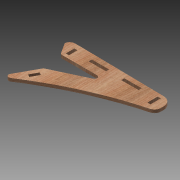
# Autodesk Inventor part: Pata con lado2
Saved by Autodesk Inventor 2015 (Build 190159000, 159)
## iProperties
Created: 2016-02-08
Part Number: Pata con lado2
Material: Wood (Birch)
Document SubType Name: Modeling
Designer: iberopuebla
Density: 0.55 g/cm^3
Appearance: Birch - Natural Polished
Author: iberopuebla
Autodesk Inventor part; units mm, degrees
ref_plane "YZ Plane" through (0, 0, 0) normal (1, 0, 0) x (0, 1, 0)
ref_plane "XZ Plane" through (0, 0, 0) normal (0, 1, 0) x (-1, 0, 0)
ref_plane "XY Plane" through (0, 0, 0) normal (0, 0, 1) x (1, 0, 0)
sketch "Sketch1" plane through (0, 0, 0) normal (0, 0, 1) x (1, 0, 0)
  arc A0 (581.4844, 252.6536) -> (22.0836, 3.3874) centre (1090.7043, -1642.4666) ccw
  line L0 (55.6223, 267.588) -> (258.6014, 267.588)
  line L1 (264.9525, 238.9989) -> (73.5785, 149.5573)
  line L2 (5.59, 332.9002) -> (42.9906, 274.4986)
  line L3 (66.787, 143.1982) -> (0.7725, 23.1982)
  arc A1 (264.9525, 238.9989) -> (258.6014, 267.588) centre (258.6014, 252.588) ccw
  arc A2 (42.9906, 274.4986) -> (55.6223, 267.588) centre (55.6223, 282.588) ccw
  arc A3 (73.5785, 149.5573) -> (66.787, 143.1982) centre (79.9296, 135.9682) ccw
  arc A4 (0.7725, 23.1982) -> (22.0836, 3.3874) centre (13.9151, 15.9682) ccw
  arc A5 (581.4844, 252.6536) -> (607.402, 286.4547) centre (572.402, 286.4547) ccw
  line L4 (77.4986, 363.1761) -> (556.5067, 355.4189)
  arc A6 (607.402, 303.6927) -> (556.5067, 355.4189) centre (555.6691, 303.6927) ccw
  line L5 (607.402, 303.6927) -> (607.402, 286.4547)
  line L6 (34.6831, 363.1761) -> (77.4986, 363.1761)
  arc A7 (34.6831, 363.1761) -> (4.8241, 336.0808) centre (34.6831, 333.1761) ccw
  arc A8 (4.8241, 336.0808) -> (5.59, 332.9002) centre (9.8006, 335.5967) ccw
  line L7 (540.6073, 347.6664) -> (560.6073, 347.6664)
  line L8 (560.6073, 347.6664) -> (560.6073, 267.6664)
  line L9 (560.6073, 267.6664) -> (540.6073, 267.6664)
  line L10 (540.6073, 267.6664) -> (540.6073, 347.6664)
  line L11 (60.6073, 346.8815) -> (80.6073, 346.8815)
  line L12 (80.6073, 346.8815) -> (80.6073, 276.8815)
  line L13 (80.6073, 276.8815) -> (60.6073, 276.8815)
  line L14 (60.6073, 276.8815) -> (60.6073, 346.8815)
  line L15 (48.4231, 57.1621) -> (96.6231, 144.7792)
  line L16 (96.6231, 144.7792) -> (114.1465, 135.1392)
  line L17 (114.1465, 135.1392) -> (65.9465, 47.5221)
  line L18 (65.9465, 47.5221) -> (48.4231, 57.1621)
  line L19 (60.6073, 470.6868) -> (560.6073, 470.6868)
  line L20 (560.6073, 470.6868) -> (560.6073, 450.6868)
  line L21 (560.6073, 450.6868) -> (60.6073, 450.6868)
  line L22 (60.6073, 450.6868) -> (60.6073, 470.6868)
  line L23 (656.5696, 347.2322) -> (-473.2183, 347.2322) construction
  point P0 (0, 0)
  point P1 (-29.0079, -30.9362)
  point P2 (47.4161, 267.588)
  point P3 (69.1456, 147.4855)
  point P4 (622.6529, 263.2389)
  dimension "d5" = 15
  dimension "d9" = 35
  dimension "d13" = 120
  dimension "d18" = 30
  dimension "d19" = 5
  dimension "d22" = 607.402
  dimension "d27" = 20
  dimension "d28" = 80
  dimension "d29" = 20
  dimension "d30" = 70
  dimension "d33" = 20
  dimension "d35" = 20
  dimension "d36" = 100
  dimension "d39" = 500
  dimension "d40" = 20
  dimension "d41" = 500
  constraints: 48 end point, 20 point on circle, 15 tangent, 9 centre point, 8 parallel, 6 point on line, 5 horizontal, 5 perpendicular, 2 equal radius
  measures "d5" radius of A1
  measures "d9" radius of A5
  measures "d13" vertical distance of L3.start L3.end
  measures "d18" radius of A7
  measures "d19" radius of A8
  measures "d22" distance from line of L5 point (0, 0)
  measures "d27" distance of L8.end L9.end
  measures "d28" distance of L7.end L8.end
  measures "d29" distance of L12.end L13.end
  measures "d30" distance of L11.end L12.end
  measures "d33" distance of L15.end L16.end
  measures "d35" distance of L17.end L15.start
  measures "d36" distance of L15.start L15.end
  measures "d39" distance of L20.end L21.end
  measures "d40" distance of L19.end L20.end
  measures "d41" distance between parallel lines of L8 L14
extrude "Extrusion1" add sketch "Sketch1" along normal blind 18 contours A0 A4 L3 A3 L1 A1 L0 A2 L2 A8 A7 L6 L4 A6 L5 A5 | L7 L8 L9 L10 | L11 L12 L13 L14 | L15 L16 L17 L18
sketch "Sketch2" plane through (0, 0, 18) normal (0, 0, 1) x (1, 0, 0)
  line L0 (76.9002, 336.193) -> (58.9002, 336.193)
  line L1 (58.9002, 336.193) -> (58.9002, 286.193)
  line L2 (58.9002, 286.193) -> (76.9002, 286.193)
  line L3 (76.9002, 286.193) -> (76.9002, 336.193)
  line L4 (540.9002, 336.193) -> (558.9002, 336.193)
  line L5 (558.9002, 336.193) -> (558.9002, 276.193)
  line L6 (558.9002, 276.193) -> (540.9002, 276.193)
  line L7 (540.9002, 276.193) -> (540.9002, 336.193)
  line L8 (79.0927, 115.5231) -> (94.8638, 106.8471)
  line L9 (54.9927, 71.7145) -> (70.7638, 63.0385)
  line L10 (70.7638, 63.0385) -> (94.8638, 106.8471)
  line L11 (54.9927, 71.7145) -> (79.0927, 115.5231)
  line L12 (9.0599, 336.193) -> (647.4361, 336.193) construction
  point P0 (0, 0)
  point P1 (67.9002, 346.193)
  dimension "d73" = 50
  dimension "d75" = 60
  dimension "d113" = 18
  dimension "d114" = 18
  dimension "d115" = 18
  dimension "d116" = 50
  constraints: 26 end point, 4 horizontal, 4 parallel, 4 perpendicular, 1 point on line
  measures "d73" distance of L1.end L0.end
  measures "d75" distance of L4.end L5.end
  measures "d113" distance between parallel lines of L3 L1
  measures "d114" distance between parallel lines of L5 L7
  measures "d115" distance between parallel lines of L10 L11
  measures "d116" distance between parallel lines of L8 L9
extrude "Extrusion2" cut sketch "Sketch2" against normal blind 18
sketch "Sketch4" plane through (0, 0, 18) normal (0, 0, 1) x (1, 0, 0)
  line L0 (58.9002, 336.193) -> (60.0316, 335.0616)
  line L1 (58.9002, 336.193) -> (60.5002, 336.193) construction
  line L2 (76.9002, 336.193) -> (75.7688, 335.0616)
  line L3 (58.9002, 286.193) -> (60.0316, 287.3243)
  line L4 (76.9002, 286.193) -> (75.7688, 287.3243)
  circle A0 centre (60.0316, 335.0616) radius 1.6
  circle A1 centre (75.7688, 335.0616) radius 1.6
  circle A2 centre (60.0316, 287.3243) radius 1.6
  circle A3 centre (75.7688, 287.3243) radius 1.6
  line L5 (79.0927, 115.5231) -> (79.5387, 113.9865)
  line L6 (54.9927, 71.7145) -> (79.0927, 115.5231) projected
  line L7 (94.8638, 106.8471) -> (93.3272, 106.4011)
  line L8 (70.7638, 63.0385) -> (70.3178, 64.5751)
  line L9 (54.9927, 71.7145) -> (56.5293, 72.1604)
  line L10 (94.8638, 106.8471) -> (79.0927, 115.5231) projected
  circle A4 centre (79.5387, 113.9865) radius 1.6
  circle A5 centre (93.3272, 106.4011) radius 1.6
  circle A6 centre (70.3178, 64.5751) radius 1.6
  circle A7 centre (56.5293, 72.1604) radius 1.6
  line L11 (540.9002, 336.193) -> (542.0316, 335.0616)
  line L12 (558.9002, 336.193) -> (557.7688, 335.0616)
  line L13 (540.9002, 276.193) -> (542.0316, 277.3243)
  line L14 (558.9002, 276.193) -> (557.7688, 277.3243)
  circle A8 centre (542.0316, 335.0616) radius 1.6
  circle A9 centre (557.7688, 335.0616) radius 1.6
  circle A10 centre (542.0316, 277.3243) radius 1.6
  circle A11 centre (557.7688, 277.3243) radius 1.6
  point P0 (0, 0)
  dimension "d80" = 1.6
  dimension "d81" = 45
  dimension "d84" = 1.6
  dimension "d85" = 1.6
  dimension "d86" = 1.6
  dimension "d88" = 3.2
  dimension "d89" = 3.2
  dimension "d90" = 3.2
  dimension "d91" = 3.2
  dimension "d92" = 1.6
  dimension "d93" = 45
  dimension "d94" = 1.6
  dimension "d95" = 1.6
  dimension "d96" = 1.6
  dimension "d97" = 45
  dimension "d98" = 45
  dimension "d99" = 3.2
  dimension "d100" = 3.2
  dimension "d101" = 3.2
  dimension "d102" = 3.2
  dimension "d103" = 1.6
  dimension "d104" = 1.6
  dimension "d106" = 1.6
  dimension "d107" = 3.2
  dimension "d108" = 3.2
  dimension "d109" = 3.2
  dimension "d110" = 3.2
  constraints: 26 end point, 12 centre point, 10 coincident, 4 perpendicular, 2 point on line, 1 equal length, 1 horizontal
  measures "d80" distance of L0.start L0.end
  measures "d81" angle of L0 L1
  measures "d84" distance of L2.start L2.end
  measures "d85" distance of L3.start L3.end
  measures "d86" distance of L4.start L4.end
  measures "d88" diameter of A0
  measures "d89" diameter of A1
  measures "d90" diameter of A2
  measures "d91" diameter of A3
  measures "d92" distance of L5.start L5.end
  measures "d93" angle of L5 L6
  measures "d94" distance of L7.start L7.end
  measures "d95" distance of L8.start L8.end
  measures "d96" distance of L6.start L9.end
  measures "d97" angle of L9 L6
  measures "d98" angle of L10 L7
  measures "d99" diameter of A4
  measures "d100" diameter of A5
  measures "d101" diameter of A6
  measures "d102" diameter of A7
  measures "d103" distance of L11.start L11.end
  measures "d104" distance of L12.start L12.end
  measures "d106" distance of L13.start L13.end
  measures "d107" diameter of A8
  measures "d108" diameter of A9
  measures "d109" diameter of A10
  measures "d110" diameter of A11
extrude "Extrusion4" cut sketch "Sketch4" against normal blind 20
sketch "Sketch5" plane through (0, 0, 18) normal (0, 0, 1) x (1, 0, 0)
  line L0 (76.9002, 276.193) -> (58.9002, 276.193)
  line L1 (58.9002, 276.193) -> (58.9002, 346.193)
  line L2 (58.9002, 346.193) -> (76.9002, 346.193)
  line L3 (76.9002, 346.193) -> (76.9002, 276.193)
  line L4 (61.163, 336.193) -> (74.6375, 336.193) projected
  line L5 (558.9002, 346.193) -> (540.9002, 346.193)
  line L6 (540.9002, 346.193) -> (540.9002, 266.193)
  line L7 (540.9002, 266.193) -> (558.9002, 266.193)
  line L8 (558.9002, 266.193) -> (558.9002, 346.193)
  line L9 (543.163, 336.193) -> (556.6375, 336.193) projected
  line L10 (-10.8781, 346.193) -> (731.1552, 346.193) construction
  line L11 (540.9002, 333.9302) -> (540.9002, 278.4557) projected
  line L12 (76.9002, 331.193) -> (540.9002, 331.193)
  line L13 (540.9002, 331.193) -> (540.9002, 313.193)
  line L14 (540.9002, 313.193) -> (76.9002, 313.193)
  line L15 (76.9002, 313.193) -> (76.9002, 331.193)
  line L16 (164.9002, 331.193) -> (164.9002, 313.193)
  line L17 (264.9002, 331.193) -> (264.9002, 313.193)
  line L18 (352.9002, 331.193) -> (352.9002, 313.193)
  line L19 (452.9002, 331.193) -> (452.9002, 313.193)
  point P0 (0, 0)
  dimension "d117" = 70
  dimension "d118" = 10
  dimension "d119" = 80
  dimension "d120" = 10
  dimension "d121" = 18
  dimension "d122" = 15
  dimension "d123" = 464
  dimension "d124" = 100
  dimension "d125" = 100
  dimension "d128" = 88
  dimension "d129" = 88
  constraints: 34 end point, 10 point on line, 7 perpendicular, 6 parallel, 5 horizontal
  measures "d117" distance of L0.end L1.end
  measures "d118" distance between parallel lines of L4 L2
  measures "d119" distance of L6.end L5.end
  measures "d120" distance between parallel lines of L9 L5
  measures "d121" distance of L12.end L13.end
  measures "d122" distance between parallel lines of L12 L10
  measures "d123" distance of L12.start L12.end
  measures "d124" distance between parallel lines of L16 L17
  measures "d125" distance between parallel lines of L19 L18
  measures "d128" distance between parallel lines of L3 L16
  measures "d129" distance between parallel lines of L13 L19
extrude "Extrusion5" cut sketch "Sketch5" against normal blind 18 contours L16 L12 L17 L14 | L18 L12 L19 L14
sketch "Sketch6" plane through (0, 0, 18) normal (0, 0, 1) x (1, 0, 0)
  line L0 (164.9002, 331.193) -> (166.0316, 330.0616)
  line L1 (164.9002, 331.193) -> (166.5002, 331.193) construction
  line L2 (164.9002, 313.193) -> (166.0316, 314.3243)
  line L3 (264.9002, 313.193) -> (263.7688, 314.3243)
  line L4 (264.9002, 331.193) -> (263.7688, 330.0616)
  circle A0 centre (166.0316, 314.3243) radius 1.6
  circle A1 centre (166.0316, 330.0616) radius 1.6
  circle A2 centre (263.7688, 330.0616) radius 1.6
  circle A3 centre (263.7688, 314.3243) radius 1.6
  line L5 (352.9002, 331.193) -> (354.0316, 330.0616)
  line L6 (352.9002, 331.193) -> (354.5002, 331.193) construction
  line L7 (352.9002, 313.193) -> (354.0316, 314.3243)
  line L8 (452.9002, 313.193) -> (451.7688, 314.3243)
  line L9 (452.9002, 331.193) -> (451.7688, 330.0616)
  circle A4 centre (451.7688, 330.0616) radius 1.6
  circle A5 centre (451.7688, 314.3243) radius 1.6
  circle A6 centre (354.0316, 330.0616) radius 1.6
  circle A7 centre (354.0316, 314.3243) radius 1.6
  point P0 (0, 0)
  dimension "d132" = 1.6
  dimension "d133" = 45
  dimension "d134" = 3.2
  dimension "d135" = 3.2
  dimension "d136" = 3.2
  dimension "d137" = 3.2
  dimension "d138" = 1.6
  dimension "d139" = 45
  dimension "d140" = 3.2
  dimension "d141" = 3.2
  dimension "d142" = 3.2
  dimension "d144" = 3.2
  constraints: 20 end point, 8 centre point, 8 coincident, 6 perpendicular, 2 equal length, 2 horizontal
  measures "d132" distance of L0.start L0.end
  measures "d133" angle of L0 L1
  measures "d134" diameter of A0
  measures "d135" diameter of A1
  measures "d136" diameter of A2
  measures "d137" diameter of A3
  measures "d138" distance of L5.start L5.end
  measures "d139" angle of L5 L6
  measures "d140" diameter of A4
  measures "d141" diameter of A5
  measures "d142" diameter of A6
  measures "d144" diameter of A7
extrude "Extrusion6" cut sketch "Sketch6" against normal blind 18
body "Solid1"
